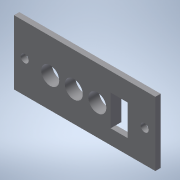
# Autodesk Inventor part: switch and led mount cap
Saved by Autodesk Inventor 2020 (Build 240168000, 168)
## iProperties
Created: 2017-06-27
Part Number: switch and led mount cap
Material: Generic
Document SubType Name: Modeling
Designer: kteo17
Density: 1 g/cm^3
Appearance: Default
Author: kteo17
## iProperties of the stored document _3DPrint.ipt
Created: 2019-06-13
Part Number: _3DPrint
Material: Generic
Document SubType Name: Modeling
Designer: cruss
Density: 1 g/cm^3
Appearance: Default
Author: cruss
Autodesk Inventor part; units mm, degrees
ref_plane "YZ Plane" through (0, 0, 0) normal (1, 0, 0) x (0, 1, 0)
ref_plane "XZ Plane" through (0, 0, 0) normal (0, 1, 0) x (-1, 0, 0)
ref_plane "XY Plane" through (0, 0, 0) normal (0, 0, 1) x (1, 0, 0)
sketch "Sketch1" plane through (0, 0, 0) normal (0, 0, 1) x (1, 0, 0)
  circle A0 centre (38.7397, 9.8403) radius 1.1906
  circle A1 centre (3.173, 9.8403) radius 1.1906
  line L0 (-0.002, 19.3653) -> (41.9147, 19.3653)
  line L1 (-0.002, 0.3153) -> (-0.002, 19.3653)
  line L2 (41.9147, 0.3153) -> (-0.002, 0.3153)
  line L3 (41.9147, 19.3653) -> (41.9147, 0.3153)
  line L4 (33.7391, 13.8091) -> (28.6591, 13.8091)
  line L5 (28.6591, 13.8091) -> (28.6591, 4.6651)
  line L6 (28.6591, 4.6651) -> (33.7391, 4.6651)
  line L7 (33.7391, 4.6651) -> (33.7391, 13.8091)
  circle A2 centre (24.7221, 9.2371) radius 2.667
  circle A3 centre (17.7371, 9.2371) radius 2.667
  circle A4 centre (10.7521, 9.2371) radius 2.667
  point P0 (0, 0)
  point P1 (33.7391, 9.2371)
  dimension "d4" = 19.05
  dimension "d5" = 3.175
  dimension "d6" = 3.175
  dimension "d34" = 2.3813
  dimension "d38" = 9.525
  dimension "d40" = 9.525
  dimension "d41" = 41.9168
  dimension "d59" = 5.334
  dimension "d60" = 5.08
  dimension "d61" = 9.144
  dimension "d62" = 0.6032
  dimension "d63" = 6.985
  dimension "d64" = 6.985
  dimension "d65" = 3.937
  dimension "d66" = 3.81
  constraints: 16 end point, 5 centre point, 3 equal radius, 3 horizontal alignment, 3 perpendicular, 2 parallel, 1 horizontal, 1 midpoint
  measures "d4" distance of L1.start L0.start
  measures "d5" distance from line of L1 A1.centre
  measures "d6" distance from line of L3 A0.centre
  measures "d34" diameter of A1
  measures "d38" distance from line of L0 A1.centre
  measures "d40" distance from line of L0 A0.centre
  measures "d41" distance between parallel lines of L3 L1
  measures "d59" diameter of A4
  measures "d60" distance of L4.start L4.end
  measures "d61" distance of L6.end L4.start
  measures "d62" vertical distance of A4.centre A1.centre
  measures "d63" distance of A3.centre A4.centre
  measures "d64" distance of A2.centre A3.centre
  measures "d65" distance from line of L5 A2.centre
  measures "d66" distance edge to line of A0 L7
extrude "Extrusion6" add sketch "Sketch1" along normal blind 1.5875
sketch "Sketch7" plane through (0, 0, 0) normal (0, 0, -1) x (-1, 0, 0)
  circle A0 centre (-24.7221, 9.2371) radius 2.667 projected
  circle A1 centre (-24.7221, 9.2371) radius 4.318
  circle A2 centre (-17.7371, 9.2371) radius 2.667 projected
  circle A3 centre (-17.7371, 9.2371) radius 4.318
  circle A4 centre (-10.7521, 9.2371) radius 2.667 projected
  circle A5 centre (-10.7521, 9.2371) radius 4.318
  line L0 (-41.9147, 19.3653) -> (0.002, 19.3653) projected
  line L1 (-34.5011, 19.3653) -> (-34.5011, 0.3153)
  line L2 (0.002, 0.3153) -> (-41.9147, 0.3153) projected
  line L3 (-7.4116, 19.3653) -> (-7.4116, 0.3153)
  line L4 (-41.9147, 19.3653) -> (0.002, 19.3653) projected
  circle A6 centre (-38.7397, 9.8403) radius 1.1906 projected
  circle A7 centre (-3.173, 9.8403) radius 1.1906 projected
  line L5 (-34.5011, 13.8091) -> (-28.0241, 13.8091)
  line L6 (-28.0241, 13.8091) -> (-28.0241, 4.6651)
  line L7 (-28.0241, 4.6651) -> (-34.5011, 4.6651)
  line L8 (-34.5011, 4.6651) -> (-34.5011, 13.8091)
  line L9 (-28.6591, 4.6651) -> (-28.6591, 13.8091) projected
  line L10 (-28.6591, 13.8091) -> (-33.7391, 13.8091) projected
  line L11 (-33.7391, 13.8091) -> (-28.6591, 13.8091)
  line L12 (-28.6591, 13.8091) -> (-28.6591, 4.6651)
  line L13 (-28.6591, 4.6651) -> (-33.7391, 4.6651)
  line L14 (-33.7391, 4.6651) -> (-33.7391, 13.8091)
  point P0 (0, 0)
  point P1 (-21.2296, 6.6978)
  point P2 (-14.2446, 6.6978)
  point P3 (-7.4116, 6.501)
  point P4 (-7.4116, 11.9731)
  point P5 (-14.2446, 11.7763)
  point P6 (-21.2296, 11.7763)
  point P7 (-28.0241, 12.0195)
  point P8 (-28.0241, 6.4546)
  dimension "d70" = 3.048
  dimension "d71" = 3.048
  dimension "d72" = 0.635
  dimension "d75" = 0
  dimension "d76" = 0
  constraints: 20 end point, 4 parallel, 3 centre point, 3 coincident, 3 perpendicular, 3 point on line, 2 equal radius, 2 horizontal, 2 tangent, 1 vertical
  measures "d70" distance edge to line of A6 L1
  measures "d71" distance edge to line of A7 L3
  measures "d72" distance between parallel lines of L6 L9
  measures "d75" distance between parallel lines of L5 L10
  measures "d76" distance between parallel lines of L13 L7
extrude "Extrusion8" add sketch "Sketch7" along normal blind 1.5875 contours A3 A1 L6 | A3 A1 | A3 A5 A2 A1 | A1 A2 A5 A3 | L6 A1 L9 | A1 L9 L5 L6 | A5 L3 A3 | A3 A5 | L6 L7 L9 A1 | L14 L7 L1 L5
body "Solid2"
